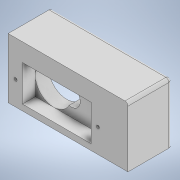
# Autodesk Inventor part: ServoMount_a
Saved by Autodesk Inventor 2022 (Build 260153000, 153)
## iProperties
Created: 2021-12-08
Part Number: ServoMount_a
Material: Generic
Document SubType Name: Modeling
Designer: dangl
Density: 1 g/cm^3
Appearance: Default
Author: dangl
Autodesk Inventor part; units mm, degrees
ref_plane "YZ Plane" through (0, 0, 0) normal (1, 0, 0) x (0, 1, 0)
ref_plane "XZ Plane" through (0, 0, 0) normal (0, 1, 0) x (-1, 0, 0)
ref_plane "XY Plane" through (0, 0, 0) normal (0, 0, 1) x (1, 0, 0)
sketch "Sketch1" plane through (0, 0, 0) normal (0, 0, 1) x (1, 0, 0)
  line L0 (0, 0) -> (-40, 0)
  line L1 (-40, 0) -> (-40, -18)
  line L2 (-40, -18) -> (0, -18)
  line L3 (0, -18) -> (0, 0)
  dimension "d0" = 40
  dimension "d1" = 18
  constraints: 8 end point, 2 parallel, 1 horizontal, 1 perpendicular
  measures "d0" distance of L0.start L0.end
  measures "d1" distance of L2.end L0.start
extrude "Extrusion1" add sketch "Sketch1" along normal blind 14.66
sketch "Sketch2" plane through (0, 0, 14.66) normal (0, 0, 1) x (1, 0, 0)
  circle A0 centre (-37.5, -12) radius 0.5
  circle A1 centre (-10, -12) radius 0.5
  line L0 (-40, -18) -> (0, -18) projected
  line L1 (-40, 0) -> (-40, -18) projected
  line L2 (-35.2, -6) -> (-12.3, -6)
  line L3 (-12.3, -6) -> (-12.3, -18)
  line L4 (-12.3, -18) -> (-35.2, -18)
  line L5 (-35.2, -18) -> (-35.2, -6)
  circle A2 centre (-29.2, -12) radius 6
  circle A3 centre (-23.2, -12) radius 3
  point P0 (0, 0)
  point P1 (-23.95, -9.0953)
  point P2 (-23.95, -14.9047)
  dimension "d4" = 1
  dimension "d5" = 1
  dimension "d6" = 6
  dimension "d7" = 6
  dimension "d8" = 27.5
  dimension "d9" = 2.5
  dimension "d10" = 12
  dimension "d11" = 4.8
  dimension "d12" = 2.3
  dimension "d17" = 6
  dimension "d18" = 6
  constraints: 8 end point, 3 centre point, 2 horizontal, 2 parallel, 1 perpendicular, 1 point on line, 3 other
  measures "d4" diameter of A0
  measures "d5" diameter of A1
  measures "d6" distance from line of L0 A0.centre
  measures "d7" distance from line of L0 A1.centre
  measures "d8" distance of A0.centre A1.centre
  measures "d9" distance from line of L1 A0.centre
  measures "d10" distance of L4.end L2.start
  measures "d11" distance between parallel lines of L1 L5
  measures "d12" distance from line of L3 A1.centre
  measures "d17" distance from line of L5 point (-29.2, -12)
  measures "d18" diameter of A3
extrude "Extrusion2" cut sketch "Sketch2" against normal blind 4.3 contours L5 A2 L0 | A2 A3 L2 L3 L0 | A2 A3 | L5 L2 A2 | A3 A2 | A2 A3
extrude "Extrusion3" cut sketch "Sketch2" against normal blind 9 contours A0 | A1
extrude "Extrusion4" cut sketch "Sketch2" against normal blind 8.75 contours A2 A3 | A3 A2 | A2 A3
sketch "Sketch3" plane through (0, 0, 5.91) normal (0, 0, 1) x (1, 0, 0)
  line L0 (-29.2, -6) -> (-12.3, -6) projected
  line L1 (-23.2, -6) -> (-41.4611, -6)
  line L2 (-41.4611, -6) -> (-41.4611, -19.254)
  line L3 (-41.4611, -19.254) -> (-23.2, -19.254)
  line L4 (-23.2, -19.254) -> (-23.2, -6)
  point P0 (0, 0)
  dimension "d21" = 23.2
  constraints: 8 end point, 2 parallel, 1 horizontal, 1 perpendicular, 1 point on line
  measures "d21" distance from line of point (0, 0) L4
extrude "Extrusion5" cut sketch "Sketch3" against normal blind 8.75
sketch "Sketch4" plane through (0, -18, 0) normal (0, -1, 0) x (1, 0, 0)
  line L0 (0, 0) -> (0, 14.66) projected
  line L1 (-23.95, 5.91) -> (-23.2, 5.91) projected
  line L2 (0, 0) -> (-23.2, 0)
  line L3 (-23.2, 0) -> (-23.2, 5.91)
  line L4 (-23.2, 5.91) -> (0, 5.91)
  line L5 (0, 5.91) -> (0, 0)
  line L6 (0, 14.66) -> (-40, 14.66) projected
  line L7 (0, 5.91) -> (-40, 5.91)
  line L8 (-40, 5.91) -> (-40, 14.66)
  line L9 (-40, 14.66) -> (0, 14.66)
  line L10 (0, 14.66) -> (0, 5.91)
  constraints: 16 end point, 4 parallel, 2 horizontal, 2 perpendicular
extrude "Extrusion6" add sketch "Sketch4" along normal blind 2
fillet "Fillet1" radius 1 3 edges at (0, -10, 0) (-20, 0, 0) (0, 0, 7.33)
equation "\"d5\" = d4"
equation "\"d6\" = 0.5 * d10"
equation "\"d7\" = d6"
equation "\"d17\" = 0.5 * d10"
body "Solid1"
